Autodesk Fusion 360 part; units mm, degrees
(part 7 of 7)
  line L817 (62.8794, -73.1457) -> (62.9313, -73.0815)
  line L818 (62.9313, -73.0815) -> (62.9798, -73.0155)
  line L819 (62.9798, -73.0155) -> (63.0231, -72.9468)
  line L820 (63.0231, -72.9468) -> (63.1792, -72.6462)
  line L821 (63.1792, -72.6462) -> (63.3657, -72.7406)
  line L822 (63.3657, -72.7406) -> (63.5541, -72.8309)
  line L823 (63.5541, -72.8309) -> (63.7444, -72.9172)
  line L824 (63.7444, -72.9172) -> (63.9366, -72.9994)
  line L825 (63.9366, -72.9994) -> (63.8066, -73.3122)
  line L826 (63.8066, -73.3122) -> (63.7819, -73.3895)
  line L827 (63.7819, -73.3895) -> (63.7625, -73.4691)
  line L828 (63.7625, -73.4691) -> (63.7466, -73.5501)
  line L829 (63.7466, -73.5501) -> (63.7337, -73.6323)
  line L830 (63.7337, -73.6323) -> (63.7234, -73.7155)
  line L831 (63.7234, -73.7155) -> (63.7154, -73.7996)
  line L832 (63.7154, -73.7996) -> (63.7096, -73.8846)
  line L833 (63.7096, -73.8846) -> (63.706, -73.9703)
  line L834 (63.706, -73.9703) -> (63.7043, -74.0567)
  line L835 (63.7043, -74.0567) -> (63.7046, -74.1438)
  line L836 (63.7046, -74.1438) -> (63.7067, -74.2315)
  line L837 (63.7067, -74.2315) -> (63.7106, -74.3197)
  line L838 (63.7106, -74.3197) -> (63.8345, -74.3665)
  line L839 (63.8345, -74.3665) -> (63.9591, -74.4119)
  line L840 (63.9591, -74.4119) -> (64.0841, -74.4557)
  line L841 (64.0841, -74.4557) -> (64.1439, -74.3906)
  line L842 (64.1439, -74.3906) -> (64.2018, -74.3248)
  line L843 (64.2018, -74.3248) -> (64.258, -74.2582)
  line L844 (64.258, -74.2582) -> (64.3123, -74.1909)
  line L845 (64.3123, -74.1909) -> (64.3645, -74.1229)
  line L846 (64.3645, -74.1229) -> (64.4147, -74.0542)
  line L847 (64.4147, -74.0542) -> (64.4627, -73.9846)
  line L848 (64.4627, -73.9846) -> (64.5083, -73.9142)
  line L849 (64.5083, -73.9142) -> (64.5512, -73.843)
  line L850 (64.5512, -73.843) -> (64.5911, -73.7707)
  line L851 (64.5911, -73.7707) -> (64.6274, -73.6973)
  line L852 (64.6274, -73.6973) -> (64.6582, -73.6221)
  line L853 (64.6582, -73.6221) -> (64.7597, -73.299)
  line L854 (64.7597, -73.299) -> (64.9597, -73.3595)
  line L855 (64.9597, -73.3595) -> (65.161, -73.4157)
  line L856 (65.161, -73.4157) -> (65.3634, -73.4677)
  line L857 (65.3634, -73.4677) -> (65.5669, -73.5153)
  line L858 (65.5669, -73.5153) -> (65.4932, -73.8459)
  line L859 (65.4932, -73.8459) -> (65.4823, -73.9263)
  line L860 (65.4823, -73.9263) -> (65.477, -74.0081)
  line L861 (65.477, -74.0081) -> (65.4755, -74.0906)
  line L862 (65.4755, -74.0906) -> (65.477, -74.1738)
  line L863 (65.477, -74.1738) -> (65.4813, -74.2575)
  line L864 (65.4813, -74.2575) -> (65.488, -74.3418)
  line L865 (65.488, -74.3418) -> (65.4971, -74.4264)
  line L866 (65.4971, -74.4264) -> (65.5084, -74.5114)
  line L867 (65.5084, -74.5114) -> (65.5218, -74.5968)
  line L868 (65.5218, -74.5968) -> (65.5371, -74.6825)
  line L869 (65.5371, -74.6825) -> (65.5544, -74.7685)
  line L870 (65.5544, -74.7685) -> (65.5736, -74.8548)
  line L871 (65.5736, -74.8548) -> (65.7038, -74.8794)
  line L872 (65.7038, -74.8794) -> (65.8343, -74.9024)
  line L873 (65.8343, -74.9024) -> (65.9651, -74.9238)
  line L874 (65.9651, -74.9238) -> (66.0126, -74.8493)
  line L875 (66.0126, -74.8493) -> (66.0583, -74.7744)
  line L876 (66.0583, -74.7744) -> (66.102, -74.6992)
  line L877 (66.102, -74.6992) -> (66.1438, -74.6235)
  line L878 (66.1438, -74.6235) -> (66.1835, -74.5474)
  line L879 (66.1835, -74.5474) -> (66.221, -74.471)
  line L880 (66.221, -74.471) -> (66.2561, -74.3942)
  line L881 (66.2561, -74.3942) -> (66.2888, -74.3169)
  line L882 (66.2888, -74.3169) -> (66.3187, -74.2393)
  line L883 (66.3187, -74.2393) -> (66.3454, -74.1612)
  line L884 (66.3454, -74.1612) -> (66.3684, -74.0826)
  line L885 (66.3684, -74.0826) -> (66.3857, -74.0032)
  line L886 (66.3857, -74.0032) -> (66.4295, -73.6674)
  line L887 (66.4295, -73.6674) -> (66.637, -73.6922)
  line L888 (66.637, -73.6922) -> (66.845, -73.7127)
  line L889 (66.845, -73.7127) -> (67.0534, -73.7287)
  line L890 (67.0534, -73.7287) -> (67.262, -73.7402)
  line L891 (67.262, -73.7402) -> (67.2469, -74.0786)
  line L892 (67.2469, -74.0786) -> (67.2501, -74.1597)
  line L893 (67.2501, -74.1597) -> (67.2591, -74.2411)
  line L894 (67.2591, -74.2411) -> (67.2719, -74.3227)
  line L895 (67.2719, -74.3227) -> (67.2879, -74.4043)
  line L896 (67.2879, -74.4043) -> (67.3066, -74.4861)
  line L897 (67.3066, -74.4861) -> (67.3279, -74.5678)
  line L898 (67.3279, -74.5678) -> (67.3515, -74.6496)
  line L899 (67.3515, -74.6496) -> (67.3774, -74.7314)
  line L900 (67.3774, -74.7314) -> (67.4054, -74.8132)
  line L901 (67.4054, -74.8132) -> (67.4354, -74.8949)
  line L902 (67.4354, -74.8949) -> (67.4674, -74.9766)
  line L903 (67.4674, -74.9766) -> (67.5012, -75.0582)
  line L904 (67.5012, -75.0582) -> (67.6337, -75.0598)
  line L905 (67.6337, -75.0598) -> (67.7663, -75.0598)
  line L906 (67.7663, -75.0598) -> (67.8988, -75.0582)
  line L907 (67.8988, -75.0582) -> (67.9326, -74.9766)
  line L908 (67.9326, -74.9766) -> (67.9646, -74.8949)
  line L909 (67.9646, -74.8949) -> (67.9946, -74.8132)
  line L910 (67.9946, -74.8132) -> (68.0226, -74.7314)
  line L911 (68.0226, -74.7314) -> (68.0485, -74.6496)
  line L912 (68.0485, -74.6496) -> (68.0721, -74.5678)
  line L913 (68.0721, -74.5678) -> (68.0934, -74.4861)
  line L914 (68.0934, -74.4861) -> (68.1121, -74.4043)
  line L915 (68.1121, -74.4043) -> (68.1281, -74.3227)
  line L916 (68.1281, -74.3227) -> (68.1409, -74.2411)
  line L917 (68.1409, -74.2411) -> (68.1499, -74.1597)
  line L918 (68.1499, -74.1597) -> (68.1531, -74.0786)
  line L919 (68.1531, -74.0786) -> (68.138, -73.7402)
  line L920 (68.138, -73.7402) -> (68.3466, -73.7287)
  line L921 (68.3466, -73.7287) -> (68.555, -73.7127)
  line L922 (68.555, -73.7127) -> (68.763, -73.6922)
  line L923 (68.763, -73.6922) -> (68.9705, -73.6674)
  line L924 (68.9705, -73.6674) -> (69.0143, -74.0032)
  line L925 (69.0143, -74.0032) -> (69.0316, -74.0826)
  line L926 (69.0316, -74.0826) -> (69.0546, -74.1612)
  line L927 (69.0546, -74.1612) -> (69.0813, -74.2393)
  line L928 (69.0813, -74.2393) -> (69.1112, -74.3169)
  line L929 (69.1112, -74.3169) -> (69.1439, -74.3942)
  line L930 (69.1439, -74.3942) -> (69.179, -74.471)
  line L931 (69.179, -74.471) -> (69.2165, -74.5474)
  line L932 (69.2165, -74.5474) -> (69.2562, -74.6235)
  line L933 (69.2562, -74.6235) -> (69.298, -74.6992)
  line L934 (69.298, -74.6992) -> (69.3417, -74.7744)
  line L935 (69.3417, -74.7744) -> (69.3874, -74.8493)
  line L936 (69.3874, -74.8493) -> (69.4349, -74.9238)
  line L937 (69.4349, -74.9238) -> (69.5657, -74.9024)
  line L938 (69.5657, -74.9024) -> (69.6962, -74.8794)
  line L939 (69.6962, -74.8794) -> (69.8264, -74.8548)
  line L940 (69.8264, -74.8548) -> (69.8456, -74.7685)
  line L941 (69.8456, -74.7685) -> (69.8629, -74.6825)
  line L942 (69.8629, -74.6825) -> (69.8782, -74.5968)
  line L943 (69.8782, -74.5968) -> (69.8916, -74.5114)
  line L944 (69.8916, -74.5114) -> (69.9029, -74.4264)
  line L945 (69.9029, -74.4264) -> (69.912, -74.3418)
  line L946 (69.912, -74.3418) -> (69.9187, -74.2575)
  line L947 (69.9187, -74.2575) -> (69.923, -74.1738)
  line L948 (69.923, -74.1738) -> (69.9245, -74.0906)
  line L949 (69.9245, -74.0906) -> (69.923, -74.0081)
  line L950 (69.923, -74.0081) -> (69.9177, -73.9263)
  line L951 (69.9177, -73.9263) -> (69.9068, -73.8459)
  line L952 (69.9068, -73.8459) -> (69.8331, -73.5153)
  line L953 (69.8331, -73.5153) -> (70.0366, -73.4677)
  line L954 (70.0366, -73.4677) -> (70.239, -73.4157)
  line L955 (70.239, -73.4157) -> (70.4403, -73.3595)
  line L956 (70.4403, -73.3595) -> (70.6403, -73.299)
  line L957 (70.6403, -73.299) -> (70.7418, -73.6221)
  line L958 (70.7418, -73.6221) -> (70.7726, -73.6973)
  line L959 (70.7726, -73.6973) -> (70.8089, -73.7707)
  line L960 (70.8089, -73.7707) -> (70.8488, -73.843)
  line L961 (70.8488, -73.843) -> (70.8917, -73.9142)
  line L962 (70.8917, -73.9142) -> (70.9373, -73.9846)
  line L963 (70.9373, -73.9846) -> (70.9853, -74.0542)
  line L964 (70.9853, -74.0542) -> (71.0355, -74.1229)
  line L965 (71.0355, -74.1229) -> (71.0877, -74.1909)
  line L966 (71.0877, -74.1909) -> (71.142, -74.2582)
  line L967 (71.142, -74.2582) -> (71.1982, -74.3248)
  line L968 (71.1982, -74.3248) -> (71.2561, -74.3906)
  line L969 (71.2561, -74.3906) -> (71.3159, -74.4557)
  line L970 (71.3159, -74.4557) -> (71.4409, -74.4119)
  line L971 (71.4409, -74.4119) -> (71.5655, -74.3665)
  line L972 (71.5655, -74.3665) -> (71.6894, -74.3197)
  line L973 (71.6894, -74.3197) -> (71.6933, -74.2315)
  line L974 (71.6933, -74.2315) -> (71.6954, -74.1438)
  line L975 (71.6954, -74.1438) -> (71.6957, -74.0567)
  line L976 (71.6957, -74.0567) -> (71.694, -73.9703)
  line L977 (71.694, -73.9703) -> (71.6904, -73.8846)
  line L978 (71.6904, -73.8846) -> (71.6846, -73.7996)
  line L979 (71.6846, -73.7996) -> (71.6766, -73.7155)
  line L980 (71.6766, -73.7155) -> (71.6663, -73.6323)
  line L981 (71.6663, -73.6323) -> (71.6534, -73.5501)
  line L982 (71.6534, -73.5501) -> (71.6375, -73.4691)
  line L983 (71.6375, -73.4691) -> (71.6181, -73.3895)
  line L984 (71.6181, -73.3895) -> (71.5934, -73.3122)
  line L985 (71.5934, -73.3122) -> (71.4634, -72.9994)
  line L986 (71.4634, -72.9994) -> (71.6556, -72.9172)
  line L987 (71.6556, -72.9172) -> (71.8459, -72.8309)
  line L988 (71.8459, -72.8309) -> (72.0343, -72.7406)
  line L989 (72.0343, -72.7406) -> (72.2208, -72.6462)
  line L990 (72.2208, -72.6462) -> (72.3769, -72.9468)
  line L991 (72.3769, -72.9468) -> (72.4202, -73.0155)
  line L992 (72.4202, -73.0155) -> (72.4687, -73.0815)
  line L993 (72.4687, -73.0815) -> (72.5206, -73.1457)
  line L994 (72.5206, -73.1457) -> (72.5752, -73.2085)
  line L995 (72.5752, -73.2085) -> (72.6323, -73.2699)
  line L996 (72.6323, -73.2699) -> (72.6917, -73.33)
  line L997 (72.6917, -73.33) -> (72.753, -73.389)
  line L998 (72.753, -73.389) -> (72.8163, -73.4469)
  line L999 (72.8163, -73.4469) -> (72.8814, -73.5038)
  line L1000 (72.8814, -73.5038) -> (72.9483, -73.5595)
  line L1001 (72.9483, -73.5595) -> (73.0168, -73.6143)
  line L1002 (73.0168, -73.6143) -> (73.087, -73.668)
  line L1003 (73.087, -73.668) -> (73.2025, -73.6032)
  line L1004 (73.2025, -73.6032) -> (73.3173, -73.5369)
  line L1005 (73.3173, -73.5369) -> (73.4312, -73.4693)
  line L1006 (73.4312, -73.4693) -> (73.4198, -73.3817)
  line L1007 (73.4198, -73.3817) -> (73.4066, -73.2949)
  line L1008 (73.4066, -73.2949) -> (73.3917, -73.2091)
  line L1009 (73.3917, -73.2091) -> (73.3751, -73.1243)
  line L1010 (73.3751, -73.1243) -> (73.3566, -73.0406)
  line L1011 (73.3566, -73.0406) -> (73.3362, -72.9579)
  line L1012 (73.3362, -72.9579) -> (73.3137, -72.8765)
  line L1013 (73.3137, -72.8765) -> (73.2891, -72.7963)
  line L1014 (73.2891, -72.7963) -> (73.2621, -72.7176)
  line L1015 (73.2621, -72.7176) -> (73.2324, -72.6406)
  line L1016 (73.2324, -72.6406) -> (73.1995, -72.5656)
  line L1017 (73.1995, -72.5656) -> (73.1617, -72.4937)
  line L1018 (73.1617, -72.4937) -> (72.9794, -72.2082)
  line L1019 (72.9794, -72.2082) -> (73.1543, -72.0939)
  line L1020 (73.1543, -72.0939) -> (73.3268, -71.9759)
  line L1021 (73.3268, -71.9759) -> (73.4967, -71.8542)
  line L1022 (73.4967, -71.8542) -> (73.6639, -71.7289)
  line L1023 (73.6639, -71.7289) -> (73.8698, -71.9978)
  line L1024 (73.8698, -71.9978) -> (73.9245, -72.0579)
  line L1025 (73.9245, -72.0579) -> (73.9837, -72.1145)
  line L1026 (73.9837, -72.1145) -> (74.0459, -72.1688)
  line L1027 (74.0459, -72.1688) -> (74.1106, -72.2211)
  line L1028 (74.1106, -72.2211) -> (74.1775, -72.2716)
  line L1029 (74.1775, -72.2716) -> (74.2464, -72.3206)
  line L1030 (74.2464, -72.3206) -> (74.3171, -72.368)
  line L1031 (74.3171, -72.368) -> (74.3895, -72.4141)
  line L1032 (74.3895, -72.4141) -> (74.4635, -72.4587)
  line L1033 (74.4635, -72.4587) -> (74.539, -72.502)
  line L1034 (74.539, -72.502) -> (74.616, -72.5441)
  line L1035 (74.616, -72.5441) -> (74.6944, -72.5848)
  line L1036 (74.6944, -72.5848) -> (74.7969, -72.5009)
  line L1037 (74.7969, -72.5009) -> (74.8984, -72.4157)
  line L1038 (74.8984, -72.4157) -> (74.9989, -72.3293)
  line L1039 (74.9989, -72.3293) -> (74.9724, -72.245)
  line L1040 (74.9724, -72.245) -> (74.9444, -72.1619)
  line L1041 (74.9444, -72.1619) -> (74.9148, -72.08)
  line L1042 (74.9148, -72.08) -> (74.8837, -71.9993)
  line L1043 (74.8837, -71.9993) -> (74.8509, -71.9201)
  line L1044 (74.8509, -71.9201) -> (74.8165, -71.8422)
  line L1045 (74.8165, -71.8422) -> (74.7802, -71.7659)
  line L1046 (74.7802, -71.7659) -> (74.7421, -71.6912)
  line L1047 (74.7421, -71.6912) -> (74.7018, -71.6184)
  line L1048 (74.7018, -71.6184) -> (74.6592, -71.5477)
  line L1049 (74.6592, -71.5477) -> (74.6137, -71.4796)
  line L1050 (74.6137, -71.4796) -> (74.564, -71.4153)
  line L1051 (74.564, -71.4153) -> (74.335, -71.1659)
  line L1052 (74.335, -71.1659) -> (74.4874, -71.0229)
  line L1053 (74.4874, -71.0229) -> (74.6367, -70.8767)
  line L1054 (74.6367, -70.8767) -> (74.7829, -70.7274)
  line L1055 (74.7829, -70.7274) -> (74.9259, -70.575)
  line L1056 (74.9259, -70.575) -> (75.1753, -70.804)
  line L1057 (75.1753, -70.804) -> (75.2396, -70.8537)
  line L1058 (75.2396, -70.8537) -> (75.3077, -70.8992)
  line L1059 (75.3077, -70.8992) -> (75.3784, -70.9418)
  line L1060 (75.3784, -70.9418) -> (75.4512, -70.9821)
  line L1061 (75.4512, -70.9821) -> (75.5259, -71.0202)
  line L1062 (75.5259, -71.0202) -> (75.6022, -71.0565)
  line L1063 (75.6022, -71.0565) -> (75.6801, -71.0909)
  line L1064 (75.6801, -71.0909) -> (75.7593, -71.1237)
  line L1065 (75.7593, -71.1237) -> (75.84, -71.1548)
  line L1066 (75.84, -71.1548) -> (75.9219, -71.1844)
  line L1067 (75.9219, -71.1844) -> (76.005, -71.2124)
  line L1068 (76.005, -71.2124) -> (76.0893, -71.2389)
  line L1069 (76.0893, -71.2389) -> (76.1757, -71.1384)
  line L1070 (76.1757, -71.1384) -> (76.2609, -71.0369)
  line L1071 (76.2609, -71.0369) -> (76.3448, -70.9344)
  line L1072 (76.3448, -70.9344) -> (76.3041, -70.856)
  line L1073 (76.3041, -70.856) -> (76.262, -70.779)
  line L1074 (76.262, -70.779) -> (76.2187, -70.7035)
  line L1075 (76.2187, -70.7035) -> (76.1741, -70.6295)
  line L1076 (76.1741, -70.6295) -> (76.128, -70.5571)
  line L1077 (76.128, -70.5571) -> (76.0806, -70.4864)
  line L1078 (76.0806, -70.4864) -> (76.0316, -70.4175)
  line L1079 (76.0316, -70.4175) -> (75.9811, -70.3506)
  line L1080 (75.9811, -70.3506) -> (75.9288, -70.2859)
  line L1081 (75.9288, -70.2859) -> (75.8745, -70.2237)
  line L1082 (75.8745, -70.2237) -> (75.8179, -70.1645)
  line L1083 (75.8179, -70.1645) -> (75.7578, -70.1098)
  line L1084 (75.7578, -70.1098) -> (75.4889, -69.9039)
  line L1085 (75.4889, -69.9039) -> (75.6142, -69.7367)
  line L1086 (75.6142, -69.7367) -> (75.7359, -69.5668)
  line L1087 (75.7359, -69.5668) -> (75.8539, -69.3943)
  line L1088 (75.8539, -69.3943) -> (75.9682, -69.2194)
  line L1089 (75.9682, -69.2194) -> (76.2537, -69.4017)
  line L1090 (76.2537, -69.4017) -> (76.3256, -69.4395)
  line L1091 (76.3256, -69.4395) -> (76.4006, -69.4724)
  line L1092 (76.4006, -69.4724) -> (76.4776, -69.5021)
  line L1093 (76.4776, -69.5021) -> (76.5563, -69.5291)
  line L1094 (76.5563, -69.5291) -> (76.6365, -69.5537)
  line L1095 (76.6365, -69.5537) -> (76.7179, -69.5762)
  line L1096 (76.7179, -69.5762) -> (76.8006, -69.5966)
  line L1097 (76.8006, -69.5966) -> (76.8843, -69.6151)
  line L1098 (76.8843, -69.6151) -> (76.9691, -69.6317)
  line L1099 (76.9691, -69.6317) -> (77.0549, -69.6466)
  line L1100 (77.0549, -69.6466) -> (77.1417, -69.6598)
  line L1101 (77.1417, -69.6598) -> (77.2293, -69.6712)
  line L1102 (77.2293, -69.6712) -> (77.2969, -69.5573)
  line L1103 (77.2969, -69.5573) -> (77.3632, -69.4425)
  line L1104 (77.3632, -69.4425) -> (77.428, -69.327)
  line L1105 (77.428, -69.327) -> (77.3743, -69.2568)
  line L1106 (77.3743, -69.2568) -> (77.3195, -69.1883)
  line L1107 (77.3195, -69.1883) -> (77.2638, -69.1214)
  line L1108 (77.2638, -69.1214) -> (77.2069, -69.0563)
  line L1109 (77.2069, -69.0563) -> (77.149, -68.993)
  line L1110 (77.149, -68.993) -> (77.09, -68.9317)
  line L1111 (77.09, -68.9317) -> (77.0299, -68.8723)
  line L1112 (77.0299, -68.8723) -> (76.9685, -68.8152)
  line L1113 (76.9685, -68.8152) -> (76.9057, -68.7606)
  line L1114 (76.9057, -68.7606) -> (76.8415, -68.7087)
  line L1115 (76.8415, -68.7087) -> (76.7755, -68.6602)
  line L1116 (76.7755, -68.6602) -> (76.7068, -68.6169)
  line L1117 (76.7068, -68.6169) -> (76.4062, -68.4608)
  line L1118 (76.4062, -68.4608) -> (76.5006, -68.2743)
  line L1119 (76.5006, -68.2743) -> (76.5909, -68.0859)
  line L1120 (76.5909, -68.0859) -> (76.6772, -67.8956)
  line L1121 (76.6772, -67.8956) -> (76.7594, -67.7034)
  line L1122 (76.7594, -67.7034) -> (77.0722, -67.8334)
  line L1123 (77.0722, -67.8334) -> (77.1495, -67.8581)
  line L1124 (77.1495, -67.8581) -> (77.2291, -67.8775)
  line L1125 (77.2291, -67.8775) -> (77.3101, -67.8934)
  line L1126 (77.3101, -67.8934) -> (77.3923, -67.9063)
  line L1127 (77.3923, -67.9063) -> (77.4755, -67.9166)
  line L1128 (77.4755, -67.9166) -> (77.5596, -67.9246)
  line L1129 (77.5596, -67.9246) -> (77.6446, -67.9304)
  line L1130 (77.6446, -67.9304) -> (77.7303, -67.934)
  line L1131 (77.7303, -67.934) -> (77.8167, -67.9357)
  line L1132 (77.8167, -67.9357) -> (77.9038, -67.9354)
  line L1133 (77.9038, -67.9354) -> (77.9915, -67.9333)
  line L1134 (77.9915, -67.9333) -> (78.0797, -67.9294)
  line L1135 (78.0797, -67.9294) -> (78.1265, -67.8055)
  line L1136 (78.1265, -67.8055) -> (78.1719, -67.6809)
  line L1137 (78.1719, -67.6809) -> (78.2157, -67.5559)
  line L1138 (78.2157, -67.5559) -> (78.1506, -67.4961)
  line L1139 (78.1506, -67.4961) -> (78.0848, -67.4382)
  line L1140 (78.0848, -67.4382) -> (78.0182, -67.382)
  line L1141 (78.0182, -67.382) -> (77.9509, -67.3277)
  line L1142 (77.9509, -67.3277) -> (77.8829, -67.2755)
  line L1143 (77.8829, -67.2755) -> (77.8142, -67.2253)
  line L1144 (77.8142, -67.2253) -> (77.7446, -67.1773)
  line L1145 (77.7446, -67.1773) -> (77.6742, -67.1317)
  line L1146 (77.6742, -67.1317) -> (77.603, -67.0888)
  line L1147 (77.603, -67.0888) -> (77.5307, -67.0489)
  line L1148 (77.5307, -67.0489) -> (77.4573, -67.0126)
  line L1149 (77.4573, -67.0126) -> (77.3821, -66.9818)
  line L1150 (77.3821, -66.9818) -> (77.059, -66.8803)
  line L1151 (77.059, -66.8803) -> (77.1195, -66.6803)
  line L1152 (77.1195, -66.6803) -> (77.1757, -66.479)
  line L1153 (77.1757, -66.479) -> (77.2277, -66.2766)
  line L1154 (77.2277, -66.2766) -> (77.2753, -66.0731)
  line L1155 (77.2753, -66.0731) -> (77.6059, -66.1468)
  line L1156 (77.6059, -66.1468) -> (77.6863, -66.1577)
  line L1157 (77.6863, -66.1577) -> (77.7681, -66.163)
  line L1158 (77.7681, -66.163) -> (77.8506, -66.1645)
  line L1159 (77.8506, -66.1645) -> (77.9338, -66.163)
  line L1160 (77.9338, -66.163) -> (78.0175, -66.1587)
  line L1161 (78.0175, -66.1587) -> (78.1018, -66.152)
  line L1162 (78.1018, -66.152) -> (78.1864, -66.1429)
  line L1163 (78.1864, -66.1429) -> (78.2714, -66.1316)
  line L1164 (78.2714, -66.1316) -> (78.3568, -66.1182)
  line L1165 (78.3568, -66.1182) -> (78.4425, -66.1029)
  line L1166 (78.4425, -66.1029) -> (78.5285, -66.0856)
  line L1167 (78.5285, -66.0856) -> (78.6148, -66.0664)
  line L1168 (78.6148, -66.0664) -> (78.6394, -65.9362)
  line L1169 (78.6394, -65.9362) -> (78.6624, -65.8057)
  line L1170 (78.6624, -65.8057) -> (78.6838, -65.6749)
  line L1171 (78.6838, -65.6749) -> (78.6093, -65.6274)
  line L1172 (78.6093, -65.6274) -> (78.5344, -65.5817)
  line L1173 (78.5344, -65.5817) -> (78.4592, -65.538)
  line L1174 (78.4592, -65.538) -> (78.3835, -65.4962)
  line L1175 (78.3835, -65.4962) -> (78.3074, -65.4565)
  line L1176 (78.3074, -65.4565) -> (78.231, -65.419)
  line L1177 (78.231, -65.419) -> (78.1542, -65.3839)
  line L1178 (78.1542, -65.3839) -> (78.0769, -65.3512)
  line L1179 (78.0769, -65.3512) -> (77.9993, -65.3213)
  line L1180 (77.9993, -65.3213) -> (77.9212, -65.2946)
  line L1181 (77.9212, -65.2946) -> (77.8426, -65.2716)
  line L1182 (77.8426, -65.2716) -> (77.7632, -65.2543)
  line L1183 (77.7632, -65.2543) -> (77.4274, -65.2105)
  line L1184 (77.4274, -65.2105) -> (77.4522, -65.003)
  line L1185 (77.4522, -65.003) -> (77.4727, -64.795)
  line L1186 (77.4727, -64.795) -> (77.4887, -64.5866)
  line L1187 (77.4887, -64.5866) -> (77.5002, -64.378)
  circle A0 centre (67.7, -63.94) radius 1.6
extrude "Extrude1''''" add sketch "Sketch1 (5)" along normal blind 2 separate body makes body 11 in component "CT dial wheel (tool body)"
component "CT sprocket pinion (tool body)" placed x (1, 0, 0) y (0, 1, 0) z (0, 0, 1) at (0, 0, 0)
component "CT idler 1" placed x (1, 0, 0) y (0, 1, 0) z (0, 0, 1) at (0, 0, 0)
component "CT idler 2" placed x (1, 0, 0) y (0, 1, 0) z (0, 0, 1) at (0, 0, 0)
component "CT idler 3" placed x (1, 0, 0) y (0, 1, 0) z (0, 0, 1) at (0, 0, 0)
component "CT dial wheel (tool body)" placed x (1, 0, 0) y (0, 1, 0) z (0, 0, 1) at (0, 0, 0)
equation "ct_module = 0.6 mm" comment "Counter train: gear module"
equation "ct_pressure_angle = 20.0 deg" comment "Counter train: pressure angle"
equation "ct_pinion_teeth = 12" comment "Counter train: teeth on every pinion"
equation "ct_wheel1_teeth = 32" comment "Counter train: idler 1 wheel (meshes sprocket pinion)"
equation "ct_wheel2_teeth = 30" comment "Counter train: idler 2 wheel"
equation "ct_wheel3_teeth = 30" comment "Counter train: idler 3 wheel"
equation "ct_wheel4_teeth = 36" comment "Counter train: dial wheel"
equation "ct_thinning = 0.125 mm" comment "Counter train: tooth thinning per gear (backlash share)"
equation "ct_pinion_shift = 0.4" comment "Counter train: pinion profile shift x (wheels get -x)"
equation "ct_pinion_tip_reduction = 0.21 mm" comment "Counter train: pinion tip shave (radial)"
equation "ct_wheel_tip_reduction = 0.04 mm" comment "Counter train: wheel tip shave (radial)"
equation "ct_sprocket_x = 73.2 mm" comment "Counter train: sprocket axis X (fixed)"
equation "ct_sprocket_y = -45.21 mm" comment "Counter train: sprocket axis Y (fixed)"
equation "ct_dial_x = 67.7 mm" comment "Counter train: dial axis X (fixed)"
equation "ct_dial_y = -63.94 mm" comment "Counter train: dial axis Y (fixed)"
equation "ct_idler1_angle = -90.74 deg" comment "Counter train: direction sprocket -> idler 1"
equation "ct_idler2_angle = -164.0 deg" comment "Counter train: direction idler 1 -> idler 2"
equation "ct_idler3_elbow = 1" comment "Counter train: idler 3 solution, 1 or -1"
equation "ct_face_width = 2.0 mm" comment "Counter train: gear face width"
equation "ct_layer_gap = 0.2 mm" comment "Counter train: axial gap between gear layers"
equation "ct_base_z = 36.8 mm" comment "Counter train: underside of idler 1 wheel"
equation "ct_clearance = 0.3 mm" comment "Counter train: minimum gap to non-meshing parts"
equation "ct_bore1 = 4.4 mm" comment "Counter train: idler 1 bore"
equation "ct_bore2 = 4.0 mm" comment "Counter train: idler 2 bore"
equation "ct_bore3 = 3.0 mm" comment "Counter train: idler 3 bore"
equation "ct_bore4 = 3.2 mm" comment "Counter train: dial wheel bore"
named bodies: "CT sprocket pinion (tool body)", "CT idler 1", "CT idler 1 pinion", "CT idler 1 wheel (1)", "CT idler 2", "CT idler 2 pinion", "CT idler 2 wheel (1)", "CT idler 3", "CT idler 3 pinion", "CT idler 3 wheel (1)", "CT dial wheel (tool body)"
